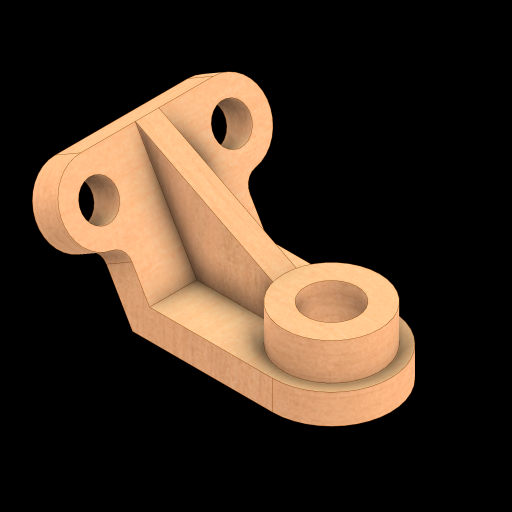
# Autodesk Inventor part: ANS9-5-BK
Saved by Autodesk Inventor 2024 (Build 280153000, 153)
## iProperties
Created: 2023-10-29
Part Number: ANS9-5-BK
Material: Wood (Cherry)
Document SubType Name: Modeling
Designer: bennk
Density: 0.63 g/cm^3
Appearance: Cherry - Natural Low Gloss
Mass: 285.995 g
Surface Area: 656.849 cm^2
Volume: 453.961 cm^3
Author: bennk
Autodesk Inventor part; units mm, degrees
ref_plane "YZ Plane" through (0, 0, 0) normal (1, 0, 0) x (0, 1, 0)
ref_plane "XZ Plane" through (0, 0, 0) normal (0, 1, 0) x (-1, 0, 0)
ref_plane "XY Plane" through (0, 0, 0) normal (0, 0, 1) x (1, 0, 0)
sketch "Sketch1" plane through (0, 0, 0) normal (0, 0, 1) x (1, 0, 0)
  line L0 (0, 0) -> (-95, 0)
  line L1 (-95, 0) -> (-142.5, 82.2724)
  line L2 (-142.5, 82.2724) -> (-125.1795, 92.2724)
  line L3 (0, 0) -> (0, 20)
  line L4 (0, 20) -> (-83.453, 20)
  line L5 (-83.453, 20) -> (-125.1795, 92.2724)
  dimension "d0" = 95
  dimension "d1" = 95
  dimension "d2" = 20
  dimension "d5" = 120
  dimension "d6" = 20
  constraints: 12 end point, 3 perpendicular, 2 horizontal
  measures "d0" distance of L0.start L0.end
  measures "d1" distance of L0.end L1.end
  measures "d2" distance of L1.end L2.end
  measures "d5" angle of L0 L1
  measures "d6" distance of L0.start L3.end
extrude "BASE" add sketch "Sketch1" along normal mid plane 80
sketch "Sketch2" plane through (-125.1795, 92.2724, 40) normal (0.8660254, 0.5, 0) x (0, 0, -1)
  arc A0 (-5, 0) -> (0, -49.4949) centre (-5, -25) ccw
  arc A1 (80, -49.4949) -> (85, 0) centre (85, -25) ccw
  line L0 (80, -142.5) -> (0, -142.5) projected
  line L1 (80, 0) -> (0, 0) projected
  line L2 (0, 0) -> (-5, 0)
  line L3 (85, 0) -> (80, 0)
  line L4 (0, 0) -> (0, -49.4949)
  line L5 (80, 0) -> (80, -49.4949)
  line L6 (80, -95) -> (80, 0) projected
  point P0 (40, -142.5)
  point P1 (40, -142.5)
  dimension "d9" = 90
  dimension "d10" = 45
  dimension "d11" = 50
  constraints: 8 end point, 4 point on circle, 4 tangent, 2 centre point, 1 equal radius, 1 horizontal, 1 midpoint, 1 perpendicular, 1 point on line
  measures "d9" distance of A1.centre A0.centre
  measures "d10" horizontal distance of A1.centre point (40, -142.5)
  measures "d11" diameter of A1
extrude "EARS" add sketch "Sketch2" against normal blind 20
fillet "Fillet1" radius 10 2 edges at (-109.0923, 44.4086, 40) (-109.0923, 44.4086, -40)
sketch "Sketch3" plane through (-83.453, 20, 40) normal (0.8660254, 0.5, 0) x (0, 0, -1)
  arc A0 (-5, 83.453) -> (-8.5714, 33.7094) centre (-5, 58.453) ccw projected
  arc A1 (88.5714, 33.7094) -> (85, 83.453) centre (85, 58.453) ccw projected
  point P0 (40, -59.047)
  constraints: 2 coincident
hole "EARHOLES" at (-112.6795, 70.6218, 45) at (-112.6795, 70.6218, -45) direction (-0.8660254, -0.5, 0) diameter 25 end through all
sketch "Sketch4" plane through (-83.453, 20, 40) normal (0, 1, 0) x (1, 0, 0)
  line L0 (83.453, 80) -> (83.453, 0) projected
  circle A0 centre (83.453, 40) radius 40
  circle A1 centre (83.453, 40) radius 17.5
  circle A2 centre (83.453, 40) radius 32.5
  dimension "d22" = 35
  dimension "d23" = 65
  constraints: 3 coincident, 2 centre point, 1 vertical alignment, 2 other
  measures "d22" diameter of A1
  measures "d23" diameter of A2
extrude "ROUNDED END" add sketch "Sketch4" against normal blind 20
extrude "RAISED BOSS" add sketch "Sketch4" along normal blind 25 contours A2 L0 A1 | L0 A1 A2
extrude "BOSS CUTOUT" cut sketch "Sketch4" along normal through all both and the other way through all contours A1 L0 | L0 A1
sketch "Sketch5" plane through (0, 0, 0) normal (0, 0, 1) x (1, 0, 0)
  line L0 (-118.9295, 81.4471) -> (-106.4295, 59.7965) projected
  line L1 (-118.9295, 81.4471) -> (-106.4295, 59.7965) projected
  line L2 (-125.1795, 92.2724) -> (-100.3077, 49.1932) projected
  line L3 (-95.359, 40.6218) -> (-100.3077, 49.1932) projected
  line L4 (-83.453, 20) -> (-95.359, 40.6218) projected
  line L5 (-95.359, 40.6218) -> (-83.453, 20) projected
  line L6 (-100.3077, 49.1932) -> (-95.359, 40.6218) projected
  line L7 (-100.3077, 49.1932) -> (-125.1795, 92.2724) projected
  line L8 (32.5, 45) -> (-32.5, 45) projected
  line L9 (-32.5, 20) -> (-32.5, 45) projected
  line L10 (-125.1795, 92.2724) -> (-32.5, 45)
  point P0 (0, 0)
  constraints: 2 end point
extrude "CONNECTING RIB" add sketch "Sketch5" along normal mid plane 16 rib yes fills toward (-89.3627, 30.3359) open curves L5 L6 L7 L10
body "Solid1"
